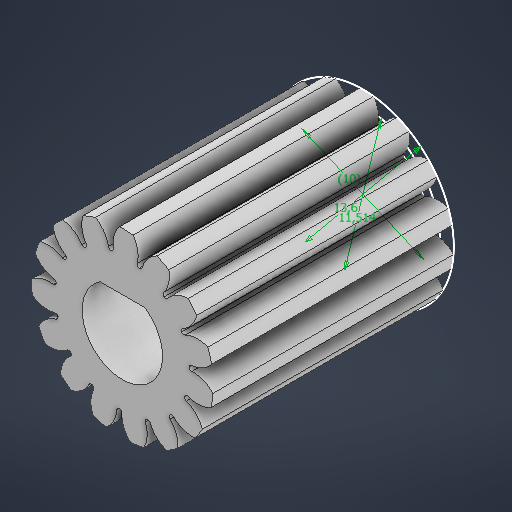
# Autodesk Inventor part: piñon
Saved by Autodesk Inventor 2025.3 (Build 293356000, 356)
## iProperties
Created: 2024-05-16
Part Number: piñon
Material: Genérico
Document SubType Name: Modeling
Designer: Jonathan Galarza
Density: 1 g/cm^3
Appearance: Valor por defecto
Author: Jonathan Galarza
Title: Eje piñon
Autodesk Inventor part; units mm, degrees
ref_plane "YZ Plane" through (0, 0, 0) normal (1, 0, 0) x (0, 1, 0)
ref_plane "XZ Plane" through (0, 0, 0) normal (0, 1, 0) x (-1, 0, 0)
ref_plane "XY Plane" through (0, 0, 0) normal (0, 0, 1) x (1, 0, 0)
sketch "Boceto1" plane through (0, 0, 0) normal (0, 0, 1) x (1, 0, 0)
  circle A0 centre (0, 0) radius 17
  dimension "d0" = 34
  constraints: 1 centre point, 1 coincident
  measures "d0" diameter of A0
extrude "Extrusión1" add sketch "Boceto1" along normal blind 1
sketch "Boceto2" plane through (0, 0, 0) normal (0, 0, -1) x (-1, 0, 0)
  point P0 (0, 0)
sketch "Boceto6" plane through (0, 0, 1) normal (0, 0, 1) x (1, 0, 0)
  arc A0 (6.6315, -1.504394) -> (6.780873, -0.509672) centre (0, 0) ccw
  circle A1 centre (0, 0) radius 5
  line L0 (0, 0) -> (6.8, 0) construction
  line L1 (0, 0) -> (6.190748, 0) construction
  arc A2 (6.780873, -0.509672) -> (4.998963, 0.101833) centre (5.298133, -1.928363) ccw
  line L2 (0, 0) -> (6.260158, 0) construction
  arc A3 (4.748577, -1.565571) -> (6.6315, -1.504394) centre (5.630835, 0.287216) ccw
  arc A4 (6.401938, 2.292421) -> (4.52536, 2.126291) centre (5.624421, 0.393298) ccw
  arc A5 (6.670069, 1.322941) -> (6.401938, 2.292421) centre (0, 0) ccw
  arc A6 (4.974816, 0.5012) -> (6.670069, 1.322941) centre (5.027203, 2.552652) ccw
  arc A7 (4.916049, 4.698133) -> (3.269282, 3.783093) centre (4.978196, 2.646954) ccw
  arc A8 (5.555323, 3.921529) -> (4.916049, 4.698133) centre (0, 0) ccw
  arc A9 (4.340864, 2.481309) -> (5.555323, 3.921529) centre (3.554321, 4.376711) ccw
  arc A10 (2.580132, 6.291496) -> (1.447915, 4.785765) centre (3.471195, 4.442927) ccw
  arc A11 (3.48001, 5.842048) -> (2.580132, 6.291496) centre (0, 0) ccw
  arc A12 (2.956338, 4.032377) -> (3.48001, 5.842048) centre (1.466865, 5.443997) ccw
  arc A13 (-0.201914, 6.797002) -> (-0.62381, 4.960934) centre (1.363993, 5.470678) ccw
  arc A14 (0.802973, 6.752424) -> (-0.201914, 6.797002) centre (0, 0) ccw
  arc A15 (1.060633, 4.886211) -> (0.802973, 6.752424) centre (-0.874226, 5.569967) ccw
  arc A16 (-2.949048, 6.127244) -> (-2.587672, 4.278312) centre (-0.979055, 5.552499) ccw
  arc A17 (-2.012906, 6.495245) -> (-2.949048, 6.127244) centre (0, 0) ccw
  arc A18 (-1.018465, 4.895174) -> (-2.012906, 6.495245) centre (-3.064154, 4.732838) ccw
  arc A19 (-5.186264, 4.39803) -> (-4.104102, 2.855932) centre (-3.152817, 4.674243) ccw
  arc A20 (-4.480736, 5.114979) -> (-5.186264, 4.39803) centre (0, 0) ccw
  arc A21 (-2.92146, 4.057717) -> (-4.480736, 5.114979) centre (-4.724263, 3.077359) ccw
  arc A22 (-6.526728, 1.908357) -> (-4.910896, 0.939735) centre (-4.781427, 2.987767) ccw
  arc A23 (-6.173805, 2.850286) -> (-6.526728, 1.908357) centre (0, 0) ccw
  arc A24 (-4.319309, 2.518644) -> (-6.173805, 2.850286) centre (-5.567504, 0.889776) ccw
  arc A25 (-6.738661, -0.911288) -> (-4.868551, -1.138951) centre (-5.583286, 0.78468) ccw
  arc A26 (-6.799367, 0.092753) -> (-6.738661, -0.911288) centre (0, 0) ccw
  arc A27 (-4.97031, 0.544075) -> (-6.799367, 0.092753) centre (-5.448072, -1.451657) ccw
  arc A28 (-5.785419, -3.573364) -> (-3.98439, -3.020702) centre (-5.419743, -1.554086) ccw
  arc A29 (-6.249257, -2.680817) -> (-5.785419, -3.573364) centre (0, 0) ccw
  arc A30 (-4.761899, -1.52457) -> (-6.249257, -2.680817) centre (-4.38662, -3.542085) ccw
  arc A31 (-3.831825, -5.617572) -> (-2.411291, -4.380146) centre (-4.319078, -3.624137) ccw
  arc A32 (-4.618594, -4.990851) -> (-3.831825, -5.617572) centre (0, 0) ccw
  arc A33 (-3.730113, -3.329603) -> (-4.618594, -4.990851) centre (-2.566681, -5.020055) ccw
  arc A34 (-1.215674, -6.690451) -> (-0.421258, -4.982223) centre (-2.471605, -5.067541) ccw
  arc A35 (-2.189334, -6.43792) -> (-1.215674, -6.690451) centre (0, 0) ccw
  arc A36 (-2.053356, -4.558918) -> (-2.189334, -6.43792) centre (-0.30294, -5.630011) ccw
  arc A37 (1.610678, -6.60649) -> (1.641614, -4.722828) centre (-0.196769, -5.634721) ccw
  arc A38 (0.618482, -6.771815) -> (1.610678, -6.60649) centre (0, 0) ccw
  arc A39 (-0.021555, -4.999954) -> (0.618482, -6.771815) centre (2.013183, -5.266488) ccw
  arc A40 (4.158529, -5.380208) -> (3.420636, -3.646814) centre (2.11209, -5.227607) ccw
  arc A41 (3.319357, -5.934802) -> (4.158529, -5.380208) centre (0, 0) ccw
  arc A42 (2.013973, -4.576452) -> (3.319357, -5.934802) centre (3.981208, -3.992341) ccw
  arc A43 (5.987333, -3.223638) -> (4.608199, -1.940232) centre (4.05575, -3.916592) ccw
  arc A44 (5.446285, -4.071607) -> (5.987333, -3.223638) centre (0, 0) ccw
  arc A45 (3.701266, -3.361641) -> (5.446285, -4.071607) centre (5.260845, -2.027882) ccw
  point P0 (-4.104102, 2.855932)
  point P1 (-4.910896, 0.939735)
  point P2 (-4.97031, 0.544075)
  point P3 (-4.868551, -1.138951)
  point P4 (-4.761899, -1.52457)
  point P5 (-3.98439, -3.020702)
  point P6 (-0.421258, -4.982223)
  point P7 (1.641614, -4.722828)
  point P8 (3.420636, -3.646814)
  point P9 (4.608199, -1.940232)
  point P10 (4.52536, 2.126291)
  point P11 (3.269282, 3.783093)
  point P12 (2.956338, 4.032377)
  point P13 (1.447915, 4.785765)
  point P14 (1.060633, 4.886211)
  point P15 (-0.62381, 4.960934)
  dimension "d46" = 10
  dimension "d17" = 360
  constraints: 90 point on circle, 45 centre point, 6 end point, 3 coincident, 3 horizontal, 152 other
extrude "Extrusión4" add sketch "Boceto6" along normal blind 19
fillet "Empalme2" radius 0.2 2 edges at (1.0606, 4.8862, 10.5) (1.4479, 4.7858, 10.5)
pattern_circular "Patrón circular2" count 15 over 360 about axis through (0, 0, 0) along (0, 0, 1) of "Empalme2"
sketch "Boceto8" plane through (0, 0, 0) normal (0, 0, -1) x (-1, 0, 0)
  circle A0 centre (0, 0) radius 17
  circle A1 centre (0, 0) radius 17
  circle A2 centre (0, 0) radius 17
  arc A3 (2.704709, 4.441949) -> (2.949048, 6.127244) centre (0.979055, 5.552499) ccw
  arc A4 (2.704709, 4.441949) -> (2.750875, 4.175247) centre (2.872891, 4.333715) ccw
  arc A5 (2.750875, 4.175247) -> (3.026386, 4.229927) centre (2.86091, 4.342256) ccw
  arc A6 (4.480736, 5.114979) -> (3.026386, 4.229927) centre (4.724263, 3.077359) ccw
  arc A7 (5.186264, 4.39803) -> (4.480736, 5.114979) centre (0, 0) ccw
  arc A8 (4.277578, 2.957819) -> (5.186264, 4.39803) centre (3.152817, 4.674243) ccw
  arc A9 (4.277578, 2.957819) -> (4.211276, 2.695396) centre (4.387197, 2.790536) ccw
  arc A10 (4.211276, 2.695396) -> (4.485207, 2.633289) centre (4.379727, 2.803212) ccw
  arc A11 (6.173805, 2.850286) -> (4.485207, 2.633289) centre (5.567504, 0.889776) ccw
  arc A12 (6.526728, 1.908357) -> (6.173805, 2.850286) centre (0, 0) ccw
  arc A13 (5.110815, 0.962254) -> (6.526728, 1.908357) centre (4.781427, 2.987767) ccw
  arc A14 (5.110815, 0.962254) -> (4.943508, 0.749486) centre (5.142917, 0.764847) ccw
  arc A15 (4.943508, 0.749486) -> (5.168496, 0.581331) centre (5.141248, 0.779466) ccw
  arc A16 (6.799367, 0.092753) -> (5.168496, 0.581331) centre (5.448072, -1.451657) ccw
  arc A17 (6.738661, -0.911288) -> (6.799367, 0.092753) centre (0, 0) ccw
  arc A18 (5.060346, -1.199693) -> (6.738661, -0.911288) centre (5.583286, 0.78468) ccw
  arc A19 (5.060346, -1.199693) -> (4.820963, -1.326016) centre (5.00938, -1.39309) ccw
  arc A20 (4.820963, -1.326016) -> (4.958104, -1.571145) centre (5.013801, -1.379057) ccw
  arc A21 (6.249257, -2.680817) -> (4.958104, -1.571145) centre (4.38662, -3.542085) ccw
  arc A22 (5.785419, -3.573364) -> (6.249257, -2.680817) centre (0, 0) ccw
  arc A23 (4.134897, -3.154202) -> (5.785419, -3.573364) centre (5.419743, -1.554086) ccw
  arc A24 (4.134897, -3.154202) -> (3.864829, -3.172238) centre (4.009676, -3.310149) ccw
  arc A25 (3.864829, -3.172238) -> (3.890412, -3.451955) centre (4.019423, -3.299128) ccw
  arc A26 (4.618594, -4.990851) -> (3.890412, -3.451955) centre (2.566681, -5.020055) ccw
  arc A27 (3.831825, -5.617572) -> (4.618594, -4.990851) centre (0, 0) ccw
  arc A28 (2.494487, -4.563321) -> (3.831825, -5.617572) centre (4.319078, -3.624137) ccw
  arc A29 (2.494487, -4.563321) -> (2.240432, -4.469951) centre (2.316662, -4.654854) ccw
  arc A30 (2.240432, -4.469951) -> (2.150031, -4.735891) centre (2.330049, -4.648749) ccw
  arc A31 (2.189334, -6.43792) -> (2.150031, -4.735891) centre (0.30294, -5.630011) ccw
  arc A32 (1.215674, -6.690451) -> (2.189334, -6.43792) centre (0, 0) ccw
  arc A33 (0.422757, -5.1834) -> (1.215674, -6.690451) centre (2.471605, -5.067541) ccw
  arc A34 (0.422757, -5.1834) -> (0.228643, -4.994769) centre (0.223076, -5.194692) ccw
  arc A35 (0.228643, -4.994769) -> (0.037891, -5.200948) centre (0.237789, -5.19456) ccw
  arc A36 (-0.618482, -6.771815) -> (0.037891, -5.200948) centre (-2.013183, -5.266488) ccw
  arc A37 (-1.610678, -6.60649) -> (-0.618482, -6.771815) centre (0, 0) ccw
  arc A38 (-1.722071, -4.907223) -> (-1.610678, -6.60649) centre (0.196769, -5.634721) ccw
  arc A39 (-1.722071, -4.907223) -> (-1.82268, -4.655947) centre (-1.909081, -4.83632) ccw
  arc A40 (-1.82268, -4.655947) -> (-2.080801, -4.766714) centre (-1.895587, -4.842184) ccw
  arc A41 (-3.319357, -5.934802) -> (-2.080801, -4.766714) centre (-3.981208, -3.992341) ccw
  arc A42 (-4.158529, -5.380208) -> (-3.319357, -5.934802) centre (0, 0) ccw
  arc A43 (-3.569137, -3.782542) -> (-4.158529, -5.380208) centre (-2.11209, -5.227607) ccw
  arc A44 (-3.569137, -3.782542) -> (-3.558845, -3.512068) centre (-3.711141, -3.641705) ccw
  arc A45 (-3.558845, -3.512068) -> (-3.839703, -3.508272) centre (-3.701199, -3.652551) ccw
  arc A46 (-5.446285, -4.071607) -> (-3.839703, -3.508272) centre (-5.260845, -2.027882) ccw
  arc A47 (-5.987333, -3.223638) -> (-5.446285, -4.071607) centre (0, 0) ccw
  arc A48 (-4.799067, -2.003825) -> (-5.987333, -3.223638) centre (-4.05575, -3.916592) ccw
  arc A49 (-4.799067, -2.003825) -> (-4.679653, -1.760921) centre (-4.871511, -1.817406) ccw
  arc A50 (-4.679653, -1.760921) -> (-4.934686, -1.643218) centre (-4.86684, -1.831358) ccw
  arc A51 (-6.6315, -1.504394) -> (-4.934686, -1.643218) centre (-5.630835, 0.287216) ccw
  arc A52 (-6.780873, -0.509672) -> (-6.6315, -1.504394) centre (0, 0) ccw
  arc A53 (-5.199195, 0.121372) -> (-6.780873, -0.509672) centre (-5.298133, -1.928363) ccw
  arc A54 (-5.199195, 0.121372) -> (-4.991307, 0.294705) centre (-5.189553, 0.321139) ccw
  arc A55 (-4.991307, 0.294705) -> (-5.176417, 0.505964) centre (-5.19096, 0.306493) ccw
  arc A56 (-6.670069, 1.322941) -> (-5.176417, 0.505964) centre (-5.027203, 2.552652) ccw
  arc A57 (-6.401938, 2.292421) -> (-6.670069, 1.322941) centre (0, 0) ccw
  arc A58 (-4.700335, 2.225582) -> (-6.401938, 2.292421) centre (-5.624421, 0.393298) ccw
  arc A59 (-4.700335, 2.225582) -> (-4.439919, 2.299374) centre (-4.610273, 2.404156) ccw
  arc A60 (-4.439919, 2.299374) -> (-4.523098, 2.567659) centre (-4.617516, 2.391349) ccw
  arc A61 (-5.555323, 3.921529) -> (-4.523098, 2.567659) centre (-3.554321, 4.376711) ccw
  arc A62 (-4.916049, 4.698133) -> (-5.555323, 3.921529) centre (0, 0) ccw
  arc A63 (-3.388744, 3.944968) -> (-4.916049, 4.698133) centre (-4.978196, 2.646954) ccw
  arc A64 (-3.388744, 3.944968) -> (-3.120828, 3.90646) centre (-3.233836, 4.071473) ccw
  arc A65 (-3.120828, 3.90646) -> (-3.087695, 4.185383) centre (-3.245661, 4.062719) ccw
  arc A66 (-3.48001, 5.842048) -> (-3.087695, 4.185383) centre (-1.466865, 5.443997) ccw
  arc A67 (-2.580132, 6.291496) -> (-3.48001, 5.842048) centre (0, 0) ccw
  arc A68 (-1.491208, 4.982234) -> (-2.580132, 6.291496) centre (-3.471195, 4.442927) ccw
  arc A69 (-1.491208, 4.982234) -> (-1.262118, 4.838084) centre (-1.298239, 5.034795) ccw
  arc A70 (-1.262118, 4.838084) -> (-1.118401, 5.079417) centre (-1.312603, 5.031608) ccw
  arc A71 (-0.802973, 6.752424) -> (-1.118401, 5.079417) centre (0.874226, 5.569967) ccw
  arc A72 (0.201914, 6.797002) -> (-0.802973, 6.752424) centre (0, 0) ccw
  arc A73 (0.664171, 5.158027) -> (0.201914, 6.797002) centre (-1.363993, 5.470678) ccw
  arc A74 (0.664171, 5.158027) -> (0.814824, 4.933159) centre (0.861836, 5.127556) ccw
  arc A75 (0.814824, 4.933159) -> (1.044275, 5.095173) centre (0.847417, 5.130486) ccw
  arc A76 (2.012906, 6.495245) -> (1.044275, 5.095173) centre (3.064154, 4.732838) ccw
  arc A77 (2.949048, 6.127244) -> (2.012906, 6.495245) centre (0, 0) ccw
  point P0 (5.032266, 16.238113)
  point P1 (0.504786, 16.992504)
  point P2 (11.201839, 12.787447)
  point P3 (7.372619, 15.31811)
  point P4 (15.434512, 7.125716)
  point P5 (12.965659, 10.995075)
  point P6 (16.998418, 0.231883)
  point P7 (16.316819, 4.770893)
  point P8 (15.623143, -6.702044)
  point P9 (16.846653, -2.278221)
  point P10 (11.546485, -12.477126)
  point P11 (14.463547, -8.933409)
  point P12 (5.473334, -16.094801)
  point P13 (9.579563, -14.04393)
  point P14 (-1.546205, -16.929538)
  point P15 (3.039185, -16.726128)
  point P16 (-8.298392, -14.837004)
  point P17 (-4.026695, -16.516226)
  point P18 (-13.615712, -10.179017)
  point P19 (-10.396324, -13.450519)
  point P20 (-16.578751, -3.760986)
  point P21 (-14.968333, -8.059095)
  point P22 (-16.675174, 3.307354)
  point P23 (-16.952182, -1.27418)
  point P24 (-13.888307, 9.803822)
  point P25 (-16.004844, 5.731052)
  point P26 (-8.700026, 14.605121)
  point P27 (-12.290124, 11.745333)
  point P28 (-2.007432, 16.881061)
  point P29 (-6.450329, 15.72874)
  constraints: 1 other
extrude "Extrusión6" cut sketch "Boceto8" against normal blind 2 contours A0 | A4 A5 A6 A7 A8 A9 A10 A11 A12 A13 A14 A15 A16 A17 A18 A19 A20 A21 A22 A23 A24 A25 A26 A27 A28 A29 A30 A31 A32 A33 A34 A35 A36 A37 A38 A39 A40 A41 A42 A43 A44 A45 A46 A47 A48 A49 A50 A51 A52 A53 A54 A55 A56 A57 A58 A59 A60 A61 A62 A63 A64 A65 A66 A67 A68 A69 A70 A71 A72 A73 A74 A75 A76 A77 A3
sketch "Boceto9" plane through (0, 0, 20) normal (0, 0, 1) x (1, 0, 0)
  circle A0 centre (0, 0) radius 3
  line L0 (0, 0) -> (0, 2.5) construction
  line L1 (0, 2.5) -> (-1.658312, 2.5)
  line L2 (0, 2.5) -> (1.658312, 2.5)
  dimension "d42" = 6
  dimension "d43" = 2.5
  constraints: 6 end point, 2 point on circle, 1 centre point, 1 coincident, 1 horizontal, 1 point on line, 1 vertical
  measures "d42" diameter of A0
  measures "d43" distance of L0.start L0.end
extrude "Extrusión7" cut sketch "Boceto9" against normal through all contours A0 L1 L2 picked at (-0.014018, -1.151904)
sketch "Boceto10" plane through (0, 0, 2) normal (0, 0, -1) x (-1, 0, 0)
  circle A0 centre (0, 0) radius 5.757075
  circle A1 centre (0, 0) radius 6.8
  arc A2 (4.943508, 0.749486) -> (5.168496, 0.581331) centre (5.141248, 0.779466) ccw
  circle A3 centre (0, 0) radius 5
  dimension "d49" = 10
  dimension "d47" = 13.6
  dimension "d48" = 11.51415
  constraints: 3 coincident, 2 centre point, 3 other
  measures "d47" diameter of A1
  measures "d48" diameter of A0
